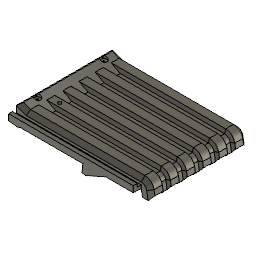
rooftile_center (Autodesk Fusion 360 design; units mm, degrees)
part number: 2026-01-25-12-36-47-508
Autodesk Fusion 360 part; units mm, degrees
sketch "tile_size" plane through (0, 0, 0) normal (0, 0, 1) x (1, 0, 0)
  line L0 (0, 0) -> (-240, 0)
  line L1 (-240, 0) -> (-240, -200)
  line L2 (-240, -200) -> (0, -200)
  line L3 (0, -200) -> (0, 0)
  dimension "d7" = 240
  dimension "d8" = 200
  constraint horizontal L0
  constraint vertical L1
  constraint horizontal L2
  constraint vertical L3
  constraint coincident L0.start L3.end
  measures "d7" distance of L0.start L0.end
  measures "d8" distance of L0.start L2.end
extrude "Extrude1" add sketch "tile_size" along normal blind 18 makes body 1
sketch "Sketch6" plane through (0, 0, 0) normal (0, 1, 0) x (1, 0, 0)
  line L0 (0, 0) -> (-240, 0)
  line L1 (-240, 0) -> (-240, -18)
  line L2 (-240, -18) -> (0, -18)
  line L3 (0, -18) -> (0, 0)
  line L4 (-240, 0) -> (71.9337, 16.3478)
  line L5 (0, 0) -> (2.2385, 12.6952)
  line L6 (-240, -18) -> (-220, -18)
  line L7 (-220, -18) -> (-222.2385, -30.6952)
  line L8 (-222.2385, -30.6952) -> (-240, -30.6952)
  line L9 (-240, -18) -> (-240, -30.6952)
  line L10 (-220, -18) -> (-253.7301, -30.6952)
  line L11 (-197.8558, -18) -> (-197.8558, -10.8) construction
  line L12 (-220, -18) -> (-200.4675, -10.6484)
  line L13 (-200.4675, -10.6484) -> (-240, -10.6484)
  dimension "d67" = 3
  dimension "d68" = 100
  dimension "d70" = 12.891
  dimension "d71" = 20
  dimension "d72" = 80
  dimension "d73" = 12.891
  dimension "d76" = 7.2
  constraint coincident L0.end L1.start
  constraint coincident L0.start L3.end
  constraint coincident L4 L5.end
  constraint coincident L1.end L2.start
  constraint coincident L2 L6.end
  constraint perpendicular L1 L8
  constraint perpendicular L8 L9
  constraint coincident L8 L10.end
  constraint coincident L2 L11.start
  constraint perpendicular L2 L11
  constraint parallel L10 L12
  constraint coincident L1 L13.end
  constraint perpendicular L1 L13
  measures "d67" angle of L0 L4
  measures "d68" angle of L0 L5
  measures "d70" distance of L0.start L5.end
  measures "d71" distance of L1.end L6.end
  measures "d72" angle of L6 L7
  measures "d73" distance of L6.end L7.end
  measures "d76" distance of L11.start L11.end
sketch "side_channels" plane through (0, 0, 0) normal (1, 0, 0) x (0, 1, 0)
  line L0 (-200, 0) -> (0, 0)
  line L1 (0, 0) -> (0, 18)
  line L2 (0, 18) -> (-200, 18)
  line L3 (-200, 18) -> (-200, 0)
  line L4 (-185, 18) -> (-185, 0)
  line L5 (-15, 18) -> (-15, 0)
  line L6 (-200, 12) -> (0, 12)
  line L7 (-200, 6) -> (0, 6)
  line L8 (-192.5, 18) -> (-192.5, 0)
  line L9 (-7.5, 18) -> (-7.5, 0)
  dimension "d13" = 15
  dimension "d14" = 15
  dimension "d15" = 6
  dimension "d16" = 6
  dimension "d18" = 7.5
  dimension "d19" = 7.5
  constraint coincident L2 L4.start
  constraint coincident L0 L4.end
  constraint perpendicular L0 L4
  constraint coincident L2 L5.start
  constraint coincident L0 L5.end
  constraint perpendicular L0 L5
  constraint coincident L3 L6.start
  constraint coincident L1 L6.end
  constraint perpendicular L1 L6
  constraint coincident L3 L7.start
  constraint coincident L1 L7.end
  constraint perpendicular L1 L7
  constraint coincident L2 L8.start
  constraint coincident L0 L8.end
  constraint perpendicular L0 L8
  constraint coincident L2 L9.start
  constraint coincident L0 L9.end
  constraint perpendicular L0 L9
  measures "d13" distance of L1 L5
  measures "d14" distance of L3 L4
  measures "d15" distance of L2 L6
  measures "d16" distance of L0 L7
  measures "d18" distance of L3 L8
  measures "d19" distance of L1 L9
extrude "Extrude2" cut sketch "side_channels" against normal up to surface (240 mm away) contours L4 L6 L7 L8 | L2 L3 L6 L8 | L0 L5 L7 L9 | L2 L4 L6 L8 | L0 L1 L7 L9 | L5 L6 L7 L9 bodies 1
sketch "grooves" plane through (0, 0, 0) normal (1, 0, 0) x (0, 1, 0)
  line L0 (-185, 18) -> (-185, 0)
  line L1 (-185, 0) -> (-177.5, 0) construction
  line L2 (-177.5, 7.2) -> (-177.5, 0) construction
  line L3 (-185, 18) -> (0, 18)
  line L4 (-177.5, 0) -> (-169.75, 0) construction
  line L5 (-169.75, 0) -> (-154.25, 0) construction
  line L6 (-169.75, 0) -> (-169.75, 18) construction
  line L7 (-154.25, 0) -> (-154.25, 18) construction
  line L8 (-177.5, 0) -> (-162, 0)
  line L9 (-162, 18) -> (-146.5, 18)
  line L10 (-154.25, 18) -> (-154.25, 10.8) construction
  line L11 (-169.75, 0) -> (-169.75, 7.2) construction
  line L12 (-175.5625, 7.2) -> (-163.9375, 7.2)
  line L13 (-160.0625, 10.8) -> (-148.4375, 10.8)
  line L14 (-177.5, 0) -> (-175.5625, 7.2)
  line L15 (-163.9375, 7.2) -> (-162, 0)
  line L16 (-160.0625, 10.8) -> (-162, 18)
  line L17 (-148.4375, 10.8) -> (-146.5, 18)
  line L18 (-131, 18) -> (-115.5, 18)
  line L19 (-129.0625, 10.8) -> (-131, 18)
  line L20 (-129.0625, 10.8) -> (-117.4375, 10.8)
  line L21 (-117.4375, 10.8) -> (-115.5, 18)
  line L22 (-144.5625, 7.2) -> (-132.9375, 7.2)
  line L23 (-132.9375, 7.2) -> (-131, 0)
  line L24 (-146.5, 0) -> (-131, 0)
  line L25 (-146.5, 0) -> (-144.5625, 7.2)
  line L26 (-100, 18) -> (-84.5, 18)
  line L27 (-98.0625, 10.8) -> (-100, 18)
  line L28 (-98.0625, 10.8) -> (-86.4375, 10.8)
  line L29 (-86.4375, 10.8) -> (-84.5, 18)
  line L30 (-113.5625, 7.2) -> (-101.9375, 7.2)
  line L31 (-101.9375, 7.2) -> (-100, 0)
  line L32 (-115.5, 0) -> (-100, 0)
  line L33 (-115.5, 0) -> (-113.5625, 7.2)
  line L34 (-69, 18) -> (-53.5, 18)
  line L35 (-67.0625, 10.8) -> (-69, 18)
  line L36 (-67.0625, 10.8) -> (-55.4375, 10.8)
  line L37 (-55.4375, 10.8) -> (-53.5, 18)
  line L38 (-82.5625, 7.2) -> (-70.9375, 7.2)
  line L39 (-70.9375, 7.2) -> (-69, 0)
  line L40 (-84.5, 0) -> (-69, 0)
  line L41 (-84.5, 0) -> (-82.5625, 7.2)
  line L42 (-38, 18) -> (-22.5, 18)
  line L43 (-36.0625, 10.8) -> (-38, 18)
  line L44 (-36.0625, 10.8) -> (-24.4375, 10.8)
  line L45 (-24.4375, 10.8) -> (-22.5, 18)
  line L46 (-51.5625, 7.2) -> (-39.9375, 7.2)
  line L47 (-39.9375, 7.2) -> (-38, 0)
  line L48 (-53.5, 0) -> (-38, 0)
  line L49 (-53.5, 0) -> (-51.5625, 7.2)
  dimension "d25" = 7.5
  dimension "d27" = 7.2
  dimension "d42" = 7.75
  dimension "d43" = 15.5
  dimension "d44" = 15.5
  dimension "d45" = 15.5
  dimension "d46" = 7.2
  dimension "d47" = 7.2
  dimension "d49" = 11.625
  dimension "d50" = 11.625
  dimension "d53" = 124
  dimension "d54" = 0
  constraint coincident L0.end L1.start
  constraint perpendicular L0 L1
  constraint vertical L2
  constraint perpendicular L2 L4
  constraint horizontal L5
  constraint coincident L3 L6.end
  constraint perpendicular L3 L6
  constraint coincident L3 L7.end
  constraint horizontal L8
  constraint parallel L8 L9
  constraint midpoint L4.end L8
  constraint midpoint L7.end L9
  constraint perpendicular L3 L7
  constraint perpendicular L9 L10
  constraint perpendicular L4 L11
  constraint horizontal L12
  constraint horizontal L13
  constraint midpoint L10.end L13
  constraint midpoint L11.end L12
  measures "d25" distance of L0.end L1.end
  measures "d27" distance of L1.end L2.start
  measures "d42" distance of L1.end L4.end
  measures "d43" distance of L4.end L5.end
  measures "d44" distance of L1.end L8.end
  measures "d45" distance of L9.start L9.end
  measures "d46" distance of L7.end L10.end
  measures "d47" distance of L4.end L11.end
  measures "d49" distance of L12.start L12.end
  measures "d50" distance of L13.start L13.end
extrude "Extrude3" cut sketch "grooves" against normal blind 220 bodies 1
sketch "Sketch4" plane through (0, 0, 0) normal (1, 0, 0) x (0, 1, 0)
  line L0 (-39.9375, 7.2) -> (-38, 0)
  line L1 (-38, 0) -> (-15, 0)
  line L2 (-15, 0) -> (-15, 12)
  line L3 (-15, 12) -> (-7.5, 12)
  line L4 (-7.5, 12) -> (-7.5, 6)
  line L5 (-7.5, 6) -> (0, 6)
  line L6 (0, 6) -> (0, 18)
  line L7 (0, 18) -> (-22.5, 18)
  line L8 (-22.5, 18) -> (-24.4375, 10.8)
  line L9 (-24.4375, 10.8) -> (-36.0625, 10.8)
  line L10 (-36.0625, 10.8) -> (-38, 18)
  line L11 (-38, 18) -> (-53.5, 18)
  line L12 (-53.5, 18) -> (-55.4375, 10.8)
  line L13 (-55.4375, 10.8) -> (-67.0625, 10.8)
  line L14 (-67.0625, 10.8) -> (-69, 18)
  line L15 (-69, 18) -> (-84.5, 18)
  line L16 (-84.5, 18) -> (-86.4375, 10.8)
  line L17 (-86.4375, 10.8) -> (-98.0625, 10.8)
  line L18 (-98.0625, 10.8) -> (-100, 18)
  line L19 (-100, 18) -> (-115.5, 18)
  line L20 (-115.5, 18) -> (-117.4375, 10.8)
  line L21 (-117.4375, 10.8) -> (-129.0625, 10.8)
  line L22 (-129.0625, 10.8) -> (-131, 18)
  line L23 (-131, 18) -> (-146.5, 18)
  line L24 (-146.5, 18) -> (-148.4375, 10.8)
  line L25 (-148.4375, 10.8) -> (-160.0625, 10.8)
  line L26 (-160.0625, 10.8) -> (-162, 18)
  line L27 (-162, 18) -> (-185, 18)
  line L28 (-185, 18) -> (-185, 6)
  line L29 (-185, 6) -> (-192.5, 6)
  line L30 (-192.5, 6) -> (-192.5, 12)
  line L31 (-192.5, 12) -> (-200, 12)
  line L32 (-200, 12) -> (-200, 0)
  line L33 (-200, 0) -> (-177.5, 0)
  line L34 (-177.5, 0) -> (-175.5625, 7.2)
  line L35 (-175.5625, 7.2) -> (-163.9375, 7.2)
  line L36 (-163.9375, 7.2) -> (-162, 0)
  line L37 (-162, 0) -> (-146.5, 0)
  line L38 (-146.5, 0) -> (-144.5625, 7.2)
  line L39 (-144.5625, 7.2) -> (-132.9375, 7.2)
  line L40 (-132.9375, 7.2) -> (-131, 0)
  line L41 (-131, 0) -> (-115.5, 0)
  line L42 (-115.5, 0) -> (-113.5625, 7.2)
  line L43 (-113.5625, 7.2) -> (-101.9375, 7.2)
  line L44 (-101.9375, 7.2) -> (-100, 0)
  line L45 (-100, 0) -> (-84.5, 0)
  line L46 (-84.5, 0) -> (-82.5625, 7.2)
  line L47 (-82.5625, 7.2) -> (-70.9375, 7.2)
  line L48 (-70.9375, 7.2) -> (-69, 0)
  line L49 (-69, 0) -> (-53.5, 0)
  line L50 (-53.5, 0) -> (-51.5625, 7.2)
  line L51 (-51.5625, 7.2) -> (-39.9375, 7.2)
  line L52 (-185, 6) -> (-185, 0)
  line L53 (-15, 0) -> (0, 0)
  line L54 (0, 0) -> (0, 6)
  constraint coincident L28.end L29.start
  constraint coincident L33 L52.end
  constraint perpendicular L33 L52
  constraint coincident L1.end L2.start
  constraint coincident L53.end L54.start
  constraint coincident L5.end L6.start
revolve "Revolve1" add sketch "Sketch4" angle 80 about axis through (0, -38, 0) along (0, 1, 0) contours L0 L1 L2 L3 L4 L5 L6 L7 L8 L9 L10 L11 L12 L13 L14 L15 L16 L17 L18 L19 L20 L21 L22 L23 L24 L25 L26 L27 L28 L33 L34 L35 L36 L37 L38 L39 L40 L41 L42 L43 L44 L45 L46 L47 L48 L49 L50 L51 L52 | L2 L3 L4 L5 L53 L54 bodies 1
extrude "Extrude4" add 1 faces at (11.8177, -12.5, 2.0838) along direction (0.173648, 0, -0.984808) blind 50 on bodies 1 bodies 1
extrude "Extrude5" cut 5 faces at (-220, -136.8125, 2.4) (-220, -167.8125, 2.4) (-220, -105.8125, 2.4) (-220, -74.8125, 2.4) (-220, -43.8125, 2.4) along direction (1, 0, 0) up to surface end surface through (-240, 0, 0) normal (-1, 0, 0) offset 0 on bodies 1 bodies 1
extrude "Extrude6" add sketch "Sketch6" against normal up to surface (185 mm away) contours L1 L2 L6 L12 L13 | L2 L6 L9 L10 bodies 1
sketch "Sketch12" plane through (-240, 0, 0) normal (-1, 0, 0) x (0, -1, 0)
  line L0 (15, 12) -> (7.5, 12)
  line L1 (7.5, 12) -> (15, 12)
  line L2 (7.5, 10.6484) -> (15, 10.6484)
  line L3 (7.5, 12) -> (15, 12)
  line L4 (15, 12) -> (15, 10.6484)
  line L5 (15, 10.6484) -> (7.5, 10.6484)
  line L6 (7.5, 10.6484) -> (7.5, 12)
  constraint horizontal L3
  constraint vertical L4
  constraint horizontal L5
  constraint vertical L6
  constraint coincident L2.end L4.end
  constraint coincident L0.end L1.start
extrude "Extrude9" cut sketch "Sketch12" against normal up to surface (240 mm away) bodies 1
move_face "OffsetFaces2" offset -0.5 3 faces at (-160, -15, 8) (-160, -12.5, 12) (-80, -7.5, 10) on bodies 1
chamfer "Chamfer2" distance 7.2 angle 45 8 edges at (-110, 0, 18) (22.0677, 0, -21.4945) (11.5702, 0, 13.7888) (-230, -185, 21.7638) (11.5702, -185, 13.7888) (22.0677, -185, -21.4945) (-110, -185, 18) (-230, 0, 21.7638) on bodies 1
chamfer "Chamfer3" distance 7 angle 45 1 edges at (-240, -92.5, 25.5275) on bodies 1
copy_body "CopyPasteBodies1" bodies 1 makes body 2
move_body "Move1" bodies 2 to x (1, 0, 0) y (0, 1, 0) z (0, 0, 1) at (214, 0, -24.5)
sketch "Sketch13" plane through (0, 0, 0) normal (0, 1, 0) x (1, 0, 0)
  line L0 (214, 24.5) -> (-26, 24.5)
  line L1 (-26, 24.5) -> (-26, 12)
  line L2 (214, 12) -> (214, 24.5)
  line L3 (0, 0) -> (-240, 0)
  line L4 (-240, 0) -> (-240, -12.5)
  line L5 (0, -12.5) -> (0, 0)
  line L6 (-240, 0) -> (-26, 24.5)
  line L7 (-240, 0) -> (-217.3322, 0)
  line L8 (-223.1439, 1.9298) -> (-240, 0)
  line L9 (-217.3322, 0) -> (-223.1439, 1.9298)
  line L10 (-53.0615, 0) -> (-91.7939, 16.9675)
  line L11 (-99.1149, 16.1294) -> (-97.2684, 0)
  line L12 (-26, 12) -> (214, 12)
  line L13 (-240, -12.5) -> (0, -12.5)
  constraint coincident L3.end L4.start
  constraint coincident L0.end L1.start
  constraint coincident L3 L7.end
  constraint coincident L6 L8.start
  constraint coincident L3 L10.start
  constraint coincident L6 L10.end
  constraint coincident L6 L11.start
  constraint coincident L3 L11.end
  constraint perpendicular L6 L11
combine "Combine1" operation cut target body 1 tool bodies 2 makes body 3 at (12.2277, -20.8125, -48.6153)
sketch "Sketch9" plane through (0, 0, 18) normal (0, 0, 1) x (-1, 0, 0)
  line L0 (220, 131) -> (220, 146.5)
  line L1 (220, 146.5) -> (0, 146.5)
  line L2 (0, 146.5) -> (0, 131)
  line L3 (0, 131) -> (220, 131)
  spline S0 degree 3 poles (200.3898, 138.549) (200.2506, 137.9883) (200.0677, 137.7037) (200.0677, 137.1029) knots 0 0 0 0 1 1 1 1
  spline S1 degree 2 poles (200.0677, 137.1029) (200.1332, 136.7228) (201.0627, 137.0425) knots 0 0 0 1 1 1
  spline S2 degree 2 poles (201.0627, 137.0425) (201.2018, 136.2929) (201.2596, 136.0918) knots 0 0 0 1 1 1
  spline S3 degree 3 poles (201.2596, 136.0918) (201.3069, 135.8906) (202.8272, 135.0636) (203.1328, 135.1307) knots 0 0 0 0 1 1 1 1
  spline S4 degree 3 poles (203.1328, 135.1307) (203.3118, 135.1866) (203.5893, 135.6949) (203.6473, 136.1538) knots 0 0 0 0 1 1 1 1
  spline S5 degree 3 poles (203.6473, 136.1538) (203.6931, 136.3935) (203.2331, 137.2652) (203.3055, 137.2807) knots 0 0 0 0 1 1 1 1
  spline S6 degree 3 poles (203.3055, 137.2807) (203.7219, 137.0891) (204.0293, 136.958) (204.1906, 137.0083) knots 0 0 0 0 1 1 1 1
  spline S7 degree 3 poles (204.1906, 137.0083) (204.5103, 137.0083) (206.4024, 138.4499) (206.4024, 138.9584) knots 0 0 0 0 1 1 1 1
  spline S8 degree 3 poles (206.4024, 138.9584) (206.4024, 139.467) (204.5103, 140.9086) (204.1906, 140.9086) knots 0 0 0 0 1 1 1 1
  spline S9 degree 3 poles (204.1906, 140.9086) (204.0296, 140.9588) (203.7222, 140.8274) (203.3055, 140.6362) knots 0 0 0 0 1 1 1 1
  spline S10 degree 3 poles (203.3055, 140.6362) (203.2331, 140.6517) (203.6931, 141.5234) (203.6473, 141.7631) knots 0 0 0 0 1 1 1 1
  spline S11 degree 3 poles (203.6473, 141.7631) (203.5893, 142.222) (203.3121, 142.7303) (203.1328, 142.7862) knots 0 0 0 0 1 1 1 1
  spline S12 degree 3 poles (203.1328, 142.7862) (202.8269, 142.853) (201.3069, 142.0262) (201.2596, 141.8251) knots 0 0 0 0 1 1 1 1
  spline S13 degree 2 poles (201.2596, 141.8251) (201.2018, 141.624) (201.0627, 140.8744) knots 0 0 0 1 1 1
  spline S14 degree 2 poles (201.0627, 140.8744) (200.1332, 141.1938) (200.0677, 140.814) knots 0 0 0 1 1 1
  spline S15 degree 3 poles (200.0677, 140.814) (200.0677, 140.2132) (200.2506, 139.7921) (200.3898, 139.2317) knots 0 0 0 0 1 1 1 1
  spline S16 degree 3 poles (200.3898, 139.2317) (199.5876, 139.2383) (198.9826, 139.9295) (198.9464, 139.8567) knots 0 0 0 0 1 1 1 1
  spline S17 degree 3 poles (198.9464, 139.8567) (198.6597, 139.7313) (198.4394, 139.4853) (198.3603, 139.1518) knots 0 0 0 0 1 1 1 1
  spline S18 degree 3 poles (198.3603, 139.1518) (198.4394, 138.6588) (199.8962, 138.4864) (200.3898, 138.5502) knots 0 0 0 0 1 1 1 1
  line L4 (200.3898, 138.5502) -> (200.3898, 138.549)
sketch "Sketch7" plane through (0, 0, 0) normal (0, 0, -1) x (1, 0, 0)
  line L0 (-240, 131) -> (-240, 115.5)
  line L1 (-240, 115.5) -> (-230, 115.5)
  line L2 (-230, 115.5) -> (-230, 26.75) construction
  line L3 (-230, 26.75) -> (-240, 26.75) construction
  line L4 (-240, 26.75) -> (-240, 115.5)
  circle A0 centre (-230, 26.75) radius 1.5
  circle A1 centre (-230, 26.75) radius 6
  line L5 (-230, 26.75) -> (-237.5842, 32.0605) construction
  line L6 (-230, 26.75) -> (-220.7413, 26.75) construction
  line L7 (-230, 26.75) -> (-237.5842, 21.4395) construction
  line L8 (-231.2287, 27.6104) -> (-231.2287, 25.8896)
  line L9 (-234.9149, 30.1915) -> (-236, 30.1915)
  line L10 (-236, 30.1915) -> (-236, 127.333)
  line L11 (-234.9149, 23.3085) -> (-236, 23.3085)
  line L12 (-236, 23.3085) -> (-236, 127.333)
  line L13 (-236.0038, 157.6905) -> (-236.0038, 152.0461)
  line L14 (-235.1319, 150.8075) -> (-236.0037, 150.8075)
  line L15 (-230.217, 154.249) -> (-220.7413, 154.249) construction
  line L16 (-236.0037, 150.8075) -> (-236.0038, 152.0461)
  line L17 (-235.1319, 157.6905) -> (-236.0038, 157.6905)
  line L18 (-230.217, 154.249) -> (-240, 154.249) construction
  circle A2 centre (-230.217, 154.249) radius 6
  line L19 (-230.217, 154.249) -> (-237.6377, 159.445) construction
  line L20 (-230.217, 154.249) -> (-237.6377, 149.053) construction
  circle A3 centre (-230.217, 154.249) radius 1.5
  line L21 (-231.4457, 155.1094) -> (-231.4457, 153.3886)
  line L22 (0, 131) -> (-240, 131)
  line L23 (-240, 115.5) -> (0, 115.5)
  line L24 (0, 115.5) -> (0, 131)
  line L25 (-240, 84.5) -> (0, 84.5)
  line L26 (0, 84.5) -> (0, 100)
  line L27 (0, 100) -> (-240, 100)
  line L28 (-240, 100) -> (-240, 84.5)
  line L29 (0, 162) -> (-240, 162)
  line L30 (-240, 162) -> (-240, 146.5)
  line L31 (-240, 146.5) -> (0, 146.5)
  line L32 (0, 146.5) -> (0, 162)
  line L33 (0, 69) -> (-240, 69)
  line L34 (-240, 69) -> (-240, 53.5)
  line L35 (-240, 53.5) -> (0, 53.5)
  line L36 (0, 53.5) -> (0, 69)
  line L37 (-240, 15.5) -> (-240, 38)
  point P0 (-236, 26.75)
  point P1 (-236.217, 154.249)
  dimension "d79" = 10
  dimension "d83" = 3
  dimension "d89" = 12
  dimension "d94" = 145
  dimension "d95" = 3
  dimension "d96" = 12
  dimension "d97" = 145
  constraint horizontal L1
  constraint vertical L2
  constraint horizontal L3
  constraint vertical L4
  constraint coincident L0.end L1.start
  constraint coincident L2.end L3.start
  constraint concentric A0 A1
  constraint horizontal L6
  constraint symmetric L3 L2.end A0.centre
  constraint symmetric L3 L5.end L7.end
  constraint coincident A0 L8.start
  constraint coincident L5 L8.start
  constraint coincident A0 L8.end
  constraint coincident L7 L8.end
  constraint coincident A1 P0
  constraint coincident L3 P0
  constraint coincident A1 L9.start
  constraint coincident L5 L9.start
  constraint parallel L3 L9
  constraint perpendicular L3 L10
  constraint coincident L7 L11.start
  constraint coincident A1 L11.start
  constraint perpendicular L0 L11
  constraint perpendicular L11 L12
  constraint horizontal L18
  constraint coincident L15.start L18.start
  constraint concentric A2 A3
  constraint horizontal L15
  constraint symmetric L15.start A2.centre L18
  constraint symmetric L20.end L19.end L18
  constraint coincident L21.start A3
  constraint coincident L21.start L19
  constraint coincident L21.end A3
  constraint coincident L21.end L20
  constraint coincident P1 A2
  constraint coincident P1 L18
  constraint coincident L17.start A2
  constraint coincident L17.start L19
  constraint parallel L17 L18
  constraint perpendicular L13 L18
  constraint coincident L14.start L20
  constraint coincident L14.start A2
  constraint perpendicular L14 L16
  constraint midpoint L3.end L37
  measures "d79" distance of L0.end L1.end
  measures "d83" diameter of A0
  measures "d89" diameter of A1
  measures "d94" angle of L5 L6
  measures "d95" diameter of A3
  measures "d96" diameter of A2
  measures "d97" angle of L15 L19
extrude "Extrude10" add sketch "Sketch13" against normal up to surface (200 mm away) contours L3 L6 L10 L11 | L3 L6 L7 L8 L9 bodies 1
sketch "Sketch15" plane through (-240, 0, 0) normal (-1, 0, 0) x (0, -1, 0)
  line L0 (184.3513, 18.5275) -> (0.6487, 18.5275)
  line L1 (0.6487, 18.5275) -> (0, 17.8344)
  line L2 (0, 17.8344) -> (0, 6)
  line L3 (0, 6) -> (7, 6)
  line L4 (7, 6) -> (7, 12.5)
  line L5 (15.5, 12.5) -> (15.5, 0)
  line L6 (15.5, 0) -> (38, 0)
  line L7 (38, 0) -> (39.9375, 7.2)
  line L8 (39.9375, 7.2) -> (51.5625, 7.2)
  line L9 (51.5625, 7.2) -> (53.5, 0)
  line L10 (53.5, 0) -> (69, 0)
  line L11 (69, 0) -> (70.9375, 7.2)
  line L12 (70.9375, 7.2) -> (82.5625, 7.2)
  line L13 (82.5625, 7.2) -> (84.5, 0)
  line L14 (84.5, 0) -> (100, 0)
  line L15 (100, 0) -> (101.9375, 7.2)
  line L16 (101.9375, 7.2) -> (113.5625, 7.2)
  line L17 (113.5625, 7.2) -> (115.5, 0)
  line L18 (115.5, 0) -> (131, 0)
  line L19 (131, 0) -> (132.9375, 7.2)
  line L20 (132.9375, 7.2) -> (144.5625, 7.2)
  line L21 (144.5625, 7.2) -> (146.5, 0)
  line L22 (146.5, 0) -> (162, 0)
  line L23 (162, 0) -> (163.9375, 7.2)
  line L24 (163.9375, 7.2) -> (175.5625, 7.2)
  line L25 (175.5625, 7.2) -> (177.5, 0)
  line L26 (177.5, 0) -> (200, 0)
  line L27 (200, 0) -> (200, 12)
  line L28 (200, 12) -> (192.5, 12)
  line L29 (192.5, 12) -> (192.5, 6)
  line L30 (192.5, 6) -> (185, 6)
  line L31 (185, 6) -> (185, 17.8344)
  line L32 (185, 17.8344) -> (184.3513, 18.5275)
  line L33 (0, 6) -> (15.5, 6)
  line L34 (15.5, 6) -> (15.5, -59.0397)
  line L35 (15.5, -59.0397) -> (0, -59.0397)
  line L36 (0, -59.0397) -> (0, 6)
  line L37 (38, 0) -> (53.5, 0)
  line L38 (53.5, 0) -> (53.5, -64.5569)
  line L39 (53.5, -64.5569) -> (38, -64.5569)
  line L40 (38, -64.5569) -> (38, 0)
  line L41 (69, 0) -> (84.5, 0)
  line L42 (84.5, 0) -> (84.5, -64.5569)
  line L43 (84.5, -64.5569) -> (69, -64.5569)
  line L44 (69, -64.5569) -> (69, 0)
  line L45 (100, 0) -> (115.5, 0)
  line L46 (115.5, 0) -> (115.5, -64.5569)
  line L47 (115.5, -64.5569) -> (100, -64.5569)
  line L48 (100, -64.5569) -> (100, 0)
  line L49 (131, 0) -> (146.5, 0)
  line L50 (146.5, 0) -> (146.5, -71.5191)
  line L51 (146.5, -71.5191) -> (131, -71.5191)
  line L52 (131, -71.5191) -> (131, 0)
  line L53 (162, 0) -> (177.5, 0)
  line L54 (177.5, 0) -> (177.5, -66.1333)
  line L55 (177.5, -66.1333) -> (162, -66.1333)
  line L56 (162, -66.1333) -> (162, 0)
  line L57 (7, 12.5) -> (15.5, 12.5)
  constraint horizontal L33
  constraint vertical L34
  constraint horizontal L35
  constraint vertical L36
  constraint coincident L2.end L3.start
  constraint horizontal L37
  constraint vertical L38
  constraint horizontal L39
  constraint vertical L40
  constraint coincident L6.end L7.start
  constraint horizontal L41
  constraint vertical L42
  constraint horizontal L43
  constraint vertical L44
  constraint coincident L10.end L11.start
  constraint horizontal L45
  constraint vertical L46
  constraint horizontal L47
  constraint vertical L48
  constraint coincident L14.end L15.start
  constraint horizontal L49
  constraint vertical L50
  constraint horizontal L51
  constraint vertical L52
  constraint coincident L18.end L19.start
  constraint horizontal L53
  constraint vertical L54
  constraint horizontal L55
  constraint vertical L56
  constraint coincident L22.end L23.start
extrude "Extrude12" cut sketch "Sketch15" against normal blind 215 contours L3 L5 L33 L34 L35 L36 | L37 L38 L39 L40 | L53 L54 L55 L56 | L41 L42 L43 L44 | L49 L50 L51 L52 | L45 L46 L47 L48 bodies 1
extrude "Extrude7" cut sketch "Sketch7" along normal blind -150 and the other way blind -20 contours A0 L8 | A3 L21 picked at (-230.2449, 27.2172) picked at (-230.0953, 153.7595) bodies 1
extrude "Extrude8" cut sketch "Sketch7" against normal blind 50 from surface at -18 contours A0 L8 | A1 | A1 L9 L12 | A1 L11 L12 | L13 L17 A2 | L13 A2 | L13 L14 L16 A2 | A3 L21 picked at (-231.2638, 26.5213) picked at (-234.5737, 154.2829) picked at (-231.4808, 154.0203) bodies 3 1
sketch "Sketch16" plane through (-240, 0, 0) normal (-1, 0, 0) x (0, -1, 0)
  line L0 (184.3513, 18.5275) -> (0.6487, 18.5275)
  line L1 (0.6487, 18.5275) -> (0, 17.8344)
  line L2 (0, 17.8344) -> (0, 6)
  line L3 (0, 6) -> (7, 6)
  line L4 (7, 6) -> (7, 12.5)
  line L5 (15.5, 12.5) -> (15.5, 0)
  line L6 (15.5, 0) -> (38, 0)
  line L7 (38, 0) -> (39.9375, 7.2)
  line L8 (39.9375, 7.2) -> (51.5625, 7.2)
  line L9 (51.5625, 7.2) -> (53.5, 0)
  line L10 (53.5, 0) -> (69, 0)
  line L11 (69, 0) -> (70.9375, 7.2)
  line L12 (70.9375, 7.2) -> (82.5625, 7.2)
  line L13 (82.5625, 7.2) -> (84.5, 0)
  line L14 (84.5, 0) -> (100, 0)
  line L15 (100, 0) -> (101.9375, 7.2)
  line L16 (101.9375, 7.2) -> (113.5625, 7.2)
  line L17 (113.5625, 7.2) -> (115.5, 0)
  line L18 (115.5, 0) -> (131, 0)
  line L19 (131, 0) -> (132.9375, 7.2)
  line L20 (132.9375, 7.2) -> (144.5625, 7.2)
  line L21 (144.5625, 7.2) -> (146.5, 0)
  line L22 (146.5, 0) -> (162, 0)
  line L23 (162, 0) -> (163.9375, 7.2)
  line L24 (163.9375, 7.2) -> (175.5625, 7.2)
  line L25 (175.5625, 7.2) -> (177.5, 0)
  line L26 (177.5, 0) -> (200, 0)
  line L27 (200, 0) -> (200, 12)
  line L28 (200, 12) -> (192.5, 12)
  line L29 (192.5, 12) -> (192.5, 6)
  line L30 (192.5, 6) -> (185, 6)
  line L31 (185, 6) -> (185, 17.8344)
  line L32 (185, 17.8344) -> (184.3513, 18.5275)
  line L33 (45.75, 7.2) -> (45.75, 18.5275)
  circle A0 centre (45.75, 11.2) radius 2.25
  line L34 (138.75, 7.2) -> (138.75, 18.5275)
  circle A1 centre (138.75, 11.2) radius 2.25
  line L35 (7, 12.5) -> (15.5, 12.5)
  dimension "d113" = 4.5
  dimension "d114" = 4
  dimension "d115" = 4.5
  dimension "d116" = 4
  constraint midpoint L8 L33.start
  constraint coincident L0 L33.end
  constraint perpendicular L0 L33
  constraint coincident L33 A0.centre
  constraint midpoint L20 L34.start
  constraint coincident L0 L34.end
  constraint perpendicular L0 L34
  constraint coincident L34 A1.centre
  measures "d113" diameter of A0
  measures "d114" distance of L33.start A0.centre
  measures "d115" diameter of A1
  measures "d116" distance of L34.start A1.centre
extrude "Extrude13" cut sketch "Sketch16" against normal blind 246 contours L34 A1 | L34 A1 | L33 A0 | L33 A0 bodies 1
extrude "Extrude14" add sketch "Sketch9" along normal blind 0.2 contours S0 S1 S2 S3 S4 S5 S6 S7 S8 S9 S10 S11 S12 S13 S14 S15 S16 S17 S18 bodies 1
hidden bodies 3
equation "height = 240 mm"
equation "width = 200 mm"
equation "thickness = 18 mm"
equation "notch_depth = thickness * 2 / 5"
equation "num_notches = 5"
equation "notch_width = notch_pair_width / 2"
equation "d7 = height"
equation "d8 = width"
equation "d9 = thickness"
equation "tile_angle = 3 deg"
equation "side_channel_width = 15 mm"
equation "d13 = side_channel_width"
equation "d14 = side_channel_width"
equation "d15 = thickness * 1 / 3"
equation "d16 = thickness * 1 / 3"
equation "generic_offset = 0.3 mm"
equation "d18 = side_channel_width / 2"
equation "d19 = side_channel_width / 2"
equation "notch_space = width - notch_side_padding * 2 - side_channel_width * 2"
equation "notch_side_padding = side_channel_width / 2"
equation "notch_pair_width = notch_space / num_notches"
equation "d25 = notch_side_padding"
equation "d27 = notch_depth"
equation "d42 = notch_pair_width / 4"
equation "d43 = notch_pair_width / 2"
equation "d44 = notch_width"
equation "d45 = notch_width"
equation "d46 = notch_depth"
equation "d47 = notch_depth"
equation "notch_small_width = notch_width * 3 / 4"
equation "d49 = notch_small_width"
equation "d50 = notch_small_width"
equation "d51 = num_notches"
equation "d53 = notch_pair_width * ( num_notches - 1 )"
equation "d57 = bend_angle"
equation "bend_angle = 80 deg"
equation "back_lip_length = 20 mm"
equation "d64 = -height + back_lip_length"
equation "d67 = tile_angle"
equation "d68 = 180 deg - bend_angle"
equation "d71 = back_lip_length"
equation "d72 = bend_angle"
equation "d73 = d70"
equation "overhang_max_angle = 40 deg"
equation "d76 = notch_depth"
equation "d79 = back_lip_length / 2"
equation "hole_size = 3 mm"
equation "d83 = hole_size"
equation "hole_counterbore_size = 12 mm"
equation "d89 = hole_counterbore_size"
equation "d90 = -thickness"
equation "d95 = hole_size"
equation "d96 = hole_counterbore_size"
equation "d98 = notch_depth"
equation "side_channel_offset = 0.5 mm"
equation "d121 = -side_channel_offset"
